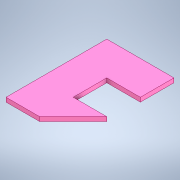
# Autodesk Inventor part: TEXAS
Saved by Autodesk Inventor 2020 (Build 240168000, 168)
## iProperties
Created: 2019-10-27
Part Number: TEXAS
Material: Generic
Document SubType Name: Modeling
Designer: Alex Zaccardelli
Density: 1 g/cm^3
Appearance: Pink
Author: Alex Zaccardelli
Autodesk Inventor part; units mm, degrees
ref_plane "YZ Plane" through (0, 0, 0) normal (1, 0, 0) x (0, 1, 0)
ref_plane "XZ Plane" through (0, 0, 0) normal (0, 1, 0) x (-1, 0, 0)
ref_plane "XY Plane" through (0, 0, 0) normal (0, 0, 1) x (1, 0, 0)
sketch "Sketch1" plane through (0, 0, 0) normal (0, 1, 0) x (-1, 0, 0)
  line L0 (6.35, -12.7) -> (-6.35, -12.7)
  line L1 (-6.35, -12.7) -> (-6.35, 12.7)
  line L2 (-6.35, 12.7) -> (6.35, 12.7)
  line L3 (6.35, 12.7) -> (6.35, -12.7)
  line L4 (6.35, -12.7) -> (-6.35, 12.7) construction
  line L5 (-6.35, -12.7) -> (6.35, 12.7) construction
  line L6 (-6.35, 0) -> (-6.35, -12.7)
  line L7 (-6.35, -12.7) -> (-19.05, -12.7)
  line L8 (-19.05, -12.7) -> (-19.05, 0)
  line L9 (-19.05, 0) -> (-6.35, 0)
  line L10 (6.35, 12.7) -> (-19.05, 12.7)
  line L11 (-6.35, 25.4) -> (6.35, 25.4)
  line L12 (6.35, 25.4) -> (6.35, 12.7)
  line L13 (-19.05, 12.7) -> (-6.35, 25.4)
  point P0 (0, 0)
  dimension "d0" = 12.7
  dimension "d1" = 25.4
  dimension "d2" = 12.7
  constraints: 28 end point, 5 parallel, 3 midpoint, 2 perpendicular, 2 point on line, 1 collinear, 1 horizontal
  measures "d0" distance of L1.end L2.end
  measures "d1" distance of L0.end L1.end
  measures "d2" distance of L0.end L7.end
extrude "Extrusion1" add sketch "Sketch1" along normal blind 1.6002
body "Solid1"
